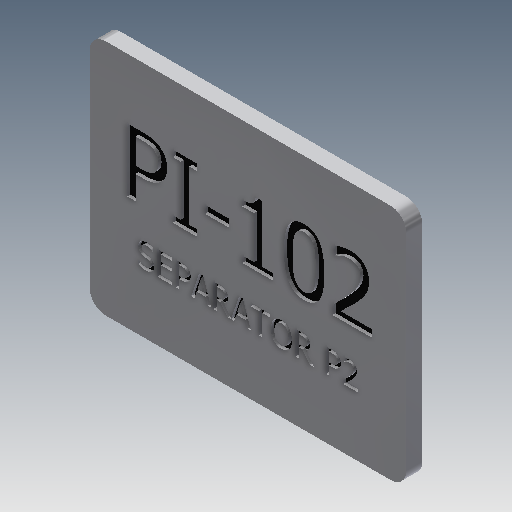
# Autodesk Inventor part: PI-102_Instrument Name Plate
Saved by Autodesk Inventor 2019.1 (Build 231200000, 200)
## iProperties
Created: 2009-08-11
Part Number: PI-102_Instrument Name Plate
Material: Polyaryletherketone Resin
Document SubType Name: Modeling
Designer: Demir Ali
Mass: 48.4669 g
Surface Area: 174.768 cm^2
Volume: 36.7173 cm^3
Density: 1.32 g/cm^3
Description: Name Plate
Stock Number: NA
Appearance: Smooth - White
Title: Purchased Part
Author: Demir Ali
Revision Number: A
Autodesk Inventor part; units mm, degrees
ref_plane "YZ Plane" through (0, 0, 0) normal (1, 0, 0) x (0, 1, 0)
ref_plane "XZ Plane" through (0, 0, 0) normal (0, 1, 0) x (-1, 0, 0)
ref_plane "XY Plane" through (0, 0, 0) normal (0, 0, 1) x (1, 0, 0)
sketch "Sketch1" plane through (0, 0, 0) normal (0, 0, 1) x (1, 0, 0)
  line L0 (-50, -37.5) -> (50, -37.5)
  line L1 (50, -37.5) -> (50, 37.5)
  line L2 (50, 37.5) -> (-50, 37.5)
  line L3 (-50, 37.5) -> (-50, -37.5)
  point P0 (0, 0)
  point P1 (50, 0)
  point P2 (0, 37.5)
  dimension "d0" = 100
  dimension "d1" = 75
  constraints: 8 end point, 2 midpoint, 2 parallel, 1 horizontal, 1 horizontal alignment, 1 perpendicular, 1 vertical alignment
  measures "d0" distance of L1.end L2.end
  measures "d1" distance of L0.end L1.end
extrude "Extrusion1" add sketch "Sketch1" along normal blind 5
sketch "Sketch2" plane through (0, 0, 5) normal (0, 0, 1) x (1, 0, 0)
  line L0 (-39.7109, 33.8079) -> (39.7109, 33.8079) construction
  line L1 (39.7109, 33.8079) -> (39.7109, -33.8079) construction
  line L2 (39.7109, -33.8079) -> (-39.7109, -33.8079) construction
  line L3 (-39.7109, -33.8079) -> (-39.7109, 33.8079) construction
  line L4 (-50, -37.5) -> (-50, 37.5) projected
  line L5 (50, -37.5) -> (-50, -37.5) projected
  line L6 (50, 37.5) -> (50, -37.5) projected
  line L7 (-50, 37.5) -> (50, 37.5) projected
  spline S0 degree 2 poles (-25.5511, 12.4253) (-25.5511, 11.1287) (-26.4749, 8.7948) (-27.3015, 7.9844) knots 0 0 0 1 2 2 2
  spline S1 degree 2 poles (-27.3015, 7.9844) (-28.3387, 6.9633) (-31.1426, 5.9099) (-33.282, 5.9099) knots 0 0 0 1 2 2 2
  line L8 (-33.282, 5.9099) -> (-35.5348, 5.9099)
  line L9 (-35.5348, 5.9099) -> (-35.5348, -1.5456)
  line L10 (-35.5348, -1.5456) -> (-38.1929, -1.5456)
  line L11 (-38.1929, -1.5456) -> (-38.1929, 18.4544)
  line L12 (-38.1929, 18.4544) -> (-33.1686, 18.4544)
  spline S2 degree 2 poles (-33.1686, 18.4544) (-31.3857, 18.4544) (-28.8898, 17.871) (-27.9336, 17.2065) knots 0 0 0 1 2 2 2
  spline S3 degree 2 poles (-27.9336, 17.2065) (-26.8152, 16.4447) (-25.5511, 14.0946) (-25.5511, 12.4253) knots 0 0 0 1 2 2 2
  spline S4 degree 2 poles (-28.3225, 12.3442) (-28.3225, 13.3815) (-29.0357, 14.905) (-29.765, 15.3912) knots 0 0 0 1 2 2 2
  spline S5 degree 2 poles (-29.765, 15.3912) (-30.3971, 15.8126) (-32.0827, 16.153) (-33.3306, 16.153) knots 0 0 0 1 2 2 2
  line L13 (-33.3306, 16.153) -> (-35.5348, 16.153)
  line L14 (-35.5348, 16.153) -> (-35.5348, 8.1789)
  line L15 (-35.5348, 8.1789) -> (-33.7196, 8.1789)
  spline S6 degree 2 poles (-33.7196, 8.1789) (-32.0989, 8.1789) (-30.1053, 8.6975) (-29.4571, 9.3783) knots 0 0 0 1 2 2 2
  spline S7 degree 2 poles (-29.4571, 9.3783) (-28.8574, 9.9779) (-28.3225, 11.388) (-28.3225, 12.3442) knots 0 0 0 1 2 2 2
  line L16 (-16.0535, -1.5456) -> (-23.8006, -1.5456)
  line L17 (-23.8006, -1.5456) -> (-23.8006, 0.4966)
  line L18 (-23.8006, 0.4966) -> (-21.2561, 0.4966)
  line L19 (-21.2561, 0.4966) -> (-21.2561, 16.4123)
  line L20 (-21.2561, 16.4123) -> (-23.8006, 16.4123)
  line L21 (-23.8006, 16.4123) -> (-23.8006, 18.4544)
  line L22 (-23.8006, 18.4544) -> (-16.0535, 18.4544)
  line L23 (-16.0535, 18.4544) -> (-16.0535, 16.4123)
  line L24 (-16.0535, 16.4123) -> (-18.5981, 16.4123)
  line L25 (-18.5981, 16.4123) -> (-18.5981, 0.4966)
  line L26 (-18.5981, 0.4966) -> (-16.0535, 0.4966)
  line L27 (-16.0535, 0.4966) -> (-16.0535, -1.5456)
  line L28 (-6.0049, 5.9909) -> (-13.5737, 5.9909)
  line L29 (-13.5737, 5.9909) -> (-13.5737, 8.422)
  line L30 (-13.5737, 8.422) -> (-6.0049, 8.422)
  line L31 (-6.0049, 8.422) -> (-6.0049, 5.9909)
  line L32 (7.9822, -1.5456) -> (-1.7747, -1.5456)
  line L33 (-1.7747, -1.5456) -> (-1.7747, 0.4966)
  line L34 (-1.7747, 0.4966) -> (1.8558, 0.4966)
  line L35 (1.8558, 0.4966) -> (1.8558, 13.9001)
  line L36 (1.8558, 13.9001) -> (-1.7747, 13.9001)
  line L37 (-1.7747, 13.9001) -> (-1.7747, 15.7316)
  spline S8 degree 2 poles (-1.7747, 15.7316) (0.2836, 15.7316) (2.2285, 16.8985) (2.3582, 18.5193) knots 0 0 0 1 2 2 2
  line L38 (2.3582, 18.5193) -> (4.4327, 18.5193)
  line L39 (4.4327, 18.5193) -> (4.4327, 0.4966)
  line L40 (4.4327, 0.4966) -> (7.9822, 0.4966)
  line L41 (7.9822, 0.4966) -> (7.9822, -1.5456)
  spline S9 degree 2 poles (24.1086, 8.4544) (24.1086, 3.0736) (20.9806, -1.967) (17.7229, -1.967) knots 0 0 0 1 2 2 2
  spline S10 degree 2 poles (17.7229, -1.967) (14.4165, -1.967) (11.3209, 3.1708) (11.3209, 8.4382) knots 0 0 0 1 2 2 2
  spline S11 degree 2 poles (11.3209, 8.4382) (11.3209, 13.8515) (14.4489, 18.8596) (17.7229, 18.8596) knots 0 0 0 1 2 2 2
  spline S12 degree 2 poles (17.7229, 18.8596) (21.013, 18.8596) (24.1086, 13.6732) (24.1086, 8.4544) knots 0 0 0 1 2 2 2
  spline S13 degree 2 poles (20.6726, 2.3604) (21.0616, 3.3491) (21.3857, 6.3961) (21.3857, 8.4544) knots 0 0 0 1 2 2 2
  spline S14 degree 2 poles (21.3857, 8.4544) (21.3857, 10.5128) (21.0616, 13.5436) (20.6564, 14.5646) knots 0 0 0 1 2 2 2
  spline S15 degree 2 poles (20.6564, 14.5646) (20.2512, 15.5857) (18.8412, 16.6392) (17.7229, 16.6392) knots 0 0 0 1 2 2 2
  spline S16 degree 2 poles (17.7229, 16.6392) (16.6045, 16.6392) (15.1621, 15.5857) (14.7407, 14.5322) knots 0 0 0 1 2 2 2
  spline S17 degree 2 poles (14.7407, 14.5322) (14.3355, 13.5112) (14.0438, 10.3993) (14.0438, 8.4382) knots 0 0 0 1 2 2 2
  spline S18 degree 2 poles (14.0438, 8.4382) (14.0438, 6.3313) (14.3031, 3.5112) (14.7245, 2.4091) knots 0 0 0 1 2 2 2
  spline S19 degree 2 poles (14.7245, 2.4091) (15.1135, 1.3718) (16.5559, 0.2535) (17.7229, 0.2535) knots 0 0 0 1 2 2 2
  spline S20 degree 2 poles (17.7229, 0.2535) (18.825, 0.2535) (20.2674, 1.3069) (20.6726, 2.3604) knots 0 0 0 1 2 2 2
  line L42 (39.0032, -1.5456) -> (26.6694, -1.5456)
  line L43 (26.6694, -1.5456) -> (26.6694, 1.2907)
  spline S21 degree 2 poles (26.6694, 1.2907) (27.9984, 2.5387) (30.3647, 4.8564) (31.4992, 6.1044) knots 0 0 0 1 2 2 2
  spline S22 degree 2 poles (31.4992, 6.1044) (33.7844, 8.6165) (35.4538, 11.6311) (35.4538, 13.2356) knots 0 0 0 1 2 2 2
  spline S23 degree 2 poles (35.4538, 13.2356) (35.4538, 14.0784) (34.9352, 15.3426) (34.4652, 15.7478) knots 0 0 0 1 2 2 2
  spline S24 degree 2 poles (34.4652, 15.7478) (33.9951, 16.153) (32.7634, 16.5582) (32.0178, 16.5582) knots 0 0 0 1 2 2 2
  spline S25 degree 2 poles (32.0178, 16.5582) (31.3047, 16.5582) (29.846, 16.2016) (29.1815, 15.9261) knots 0 0 0 1 2 2 2
  spline S26 degree 2 poles (29.1815, 15.9261) (28.6143, 15.6992) (27.5608, 15.0509) (27.2366, 14.824) knots 0 0 0 1 2 2 2
  line L44 (27.2366, 14.824) -> (27.0908, 14.824)
  line L45 (27.0908, 14.824) -> (27.0908, 17.6765)
  spline S27 degree 2 poles (27.0908, 17.6765) (27.9173, 18.0817) (30.8833, 18.8758) (32.2123, 18.8758) knots 0 0 0 1 2 2 2
  spline S28 degree 2 poles (32.2123, 18.8758) (35.0162, 18.8758) (38.1767, 15.9099) (38.1767, 13.3815) knots 0 0 0 1 2 2 2
  spline S29 degree 2 poles (38.1767, 13.3815) (38.1767, 12.1984) (37.6256, 10.221) (37.1394, 9.3783) knots 0 0 0 1 2 2 2
  spline S30 degree 2 poles (37.1394, 9.3783) (36.6532, 8.5031) (35.2431, 6.7851) (34.4652, 5.9585) knots 0 0 0 1 2 2 2
  spline S31 degree 2 poles (34.4652, 5.9585) (33.201, 4.5809) (30.1053, 1.6311) (29.1815, 0.7721) knots 0 0 0 1 2 2 2
  line L46 (29.1815, 0.7721) -> (39.0032, 0.7721)
  line L47 (39.0032, 0.7721) -> (39.0032, -1.5456)
  spline S32 degree 2 poles (-32.2761, -18.8515) (-33.0906, -18.8515) (-34.2332, -18.5112) (-34.7376, -18.268) knots 0 0 0 1 2 2 2
  line L48 (-34.7376, -18.268) -> (-34.7376, -17.016)
  line L49 (-34.7376, -17.016) -> (-34.6647, -17.016)
  spline S33 degree 2 poles (-34.6647, -17.016) (-34.1724, -17.4779) (-32.9265, -17.9885) (-32.3491, -17.9885) knots 0 0 0 1 2 2 2
  spline S34 degree 2 poles (-32.3491, -17.9885) (-31.5225, -17.9885) (-30.6777, -17.3017) (-30.6777, -16.7364) knots 0 0 0 1 2 2 2
  spline S35 degree 2 poles (-30.6777, -16.7364) (-30.6777, -16.2867) (-31.1214, -15.7275) (-31.6015, -15.5877) knots 0 0 0 1 2 2 2
  spline S36 degree 2 poles (-31.6015, -15.5877) (-31.9479, -15.4905) (-32.5253, -15.3568) (-32.9568, -15.2474) knots 0 0 0 1 2 2 2
  spline S37 degree 2 poles (-32.9568, -15.2474) (-33.3458, -15.1441) (-33.9597, -14.8341) (-34.1967, -14.5849) knots 0 0 0 1 2 2 2
  spline S38 degree 2 poles (-34.1967, -14.5849) (-34.4277, -14.3357) (-34.6829, -13.6672) (-34.6829, -13.2296) knots 0 0 0 1 2 2 2
  spline S39 degree 2 poles (-34.6829, -13.2296) (-34.6829, -12.3179) (-33.2607, -11.0841) (-32.1607, -11.0841) knots 0 0 0 1 2 2 2
  spline S40 degree 2 poles (-32.1607, -11.0841) (-31.5286, -11.0841) (-30.4103, -11.3333) (-29.9301, -11.5703) knots 0 0 0 1 2 2 2
  line L50 (-29.9301, -11.5703) -> (-29.9301, -12.7616)
  line L51 (-29.9301, -12.7616) -> (-30.003, -12.7616)
  spline S41 degree 2 poles (-30.003, -12.7616) (-30.3616, -12.4334) (-31.4799, -11.9471) (-32.0938, -11.9471) knots 0 0 0 1 2 2 2
  spline S42 degree 2 poles (-32.0938, -11.9471) (-32.7867, -11.9471) (-33.6436, -12.5975) (-33.6436, -13.1262) knots 0 0 0 1 2 2 2
  spline S43 degree 2 poles (-33.6436, -13.1262) (-33.6436, -13.6003) (-33.1392, -14.1655) (-32.6651, -14.2932) knots 0 0 0 1 2 2 2
  spline S44 degree 2 poles (-32.6651, -14.2932) (-32.3491, -14.3783) (-31.4313, -14.5971) (-31.1274, -14.6882) knots 0 0 0 1 2 2 2
  spline S45 degree 2 poles (-31.1274, -14.6882) (-30.3556, -14.9253) (-29.6384, -15.8795) (-29.6384, -16.5784) knots 0 0 0 1 2 2 2
  spline S46 degree 2 poles (-29.6384, -16.5784) (-29.6384, -17.0221) (-29.997, -17.873) (-30.3191, -18.1708) knots 0 0 0 1 2 2 2
  spline S47 degree 2 poles (-30.3191, -18.1708) (-30.6777, -18.499) (-31.5893, -18.8515) (-32.2761, -18.8515) knots 0 0 0 1 2 2 2
  line L52 (-28.6234, -18.7178) -> (-28.6234, -11.2178)
  line L53 (-28.6234, -11.2178) -> (-23.9313, -11.2178)
  line L54 (-23.9313, -11.2178) -> (-23.9313, -12.1052)
  line L55 (-23.9313, -12.1052) -> (-27.6266, -12.1052)
  line L56 (-27.6266, -12.1052) -> (-27.6266, -14.1595)
  line L57 (-27.6266, -14.1595) -> (-24.1805, -14.1595)
  line L58 (-24.1805, -14.1595) -> (-24.1805, -15.0468)
  line L59 (-24.1805, -15.0468) -> (-27.6266, -15.0468)
  line L60 (-27.6266, -15.0468) -> (-27.6266, -17.8304)
  line L61 (-27.6266, -17.8304) -> (-23.9313, -17.8304)
  line L62 (-23.9313, -17.8304) -> (-23.9313, -18.7178)
  line L63 (-23.9313, -18.7178) -> (-28.6234, -18.7178)
  spline S48 degree 2 poles (-18.0966, -13.4787) (-18.0966, -13.965) (-18.4431, -14.8402) (-18.753, -15.1441) knots 0 0 0 1 2 2 2
  spline S49 degree 2 poles (-18.753, -15.1441) (-19.142, -15.527) (-20.1935, -15.922) (-20.9957, -15.922) knots 0 0 0 1 2 2 2
  line L64 (-20.9957, -15.922) -> (-21.8406, -15.922)
  line L65 (-21.8406, -15.922) -> (-21.8406, -18.7178)
  line L66 (-21.8406, -18.7178) -> (-22.8373, -18.7178)
  line L67 (-22.8373, -18.7178) -> (-22.8373, -11.2178)
  line L68 (-22.8373, -11.2178) -> (-20.9532, -11.2178)
  spline S50 degree 2 poles (-20.9532, -11.2178) (-20.2846, -11.2178) (-19.3487, -11.4366) (-18.9901, -11.6858) knots 0 0 0 1 2 2 2
  spline S51 degree 2 poles (-18.9901, -11.6858) (-18.5707, -11.9714) (-18.0966, -12.8527) (-18.0966, -13.4787) knots 0 0 0 1 2 2 2
  spline S52 degree 2 poles (-19.1359, -13.5091) (-19.1359, -13.1202) (-19.4034, -12.5488) (-19.6769, -12.3665) knots 0 0 0 1 2 2 2
  spline S53 degree 2 poles (-19.6769, -12.3665) (-19.9139, -12.2085) (-20.546, -12.0808) (-21.014, -12.0808) knots 0 0 0 1 2 2 2
  line L69 (-21.014, -12.0808) -> (-21.8406, -12.0808)
  line L70 (-21.8406, -12.0808) -> (-21.8406, -15.0711)
  line L71 (-21.8406, -15.0711) -> (-21.1598, -15.0711)
  spline S54 degree 2 poles (-21.1598, -15.0711) (-20.5521, -15.0711) (-19.8045, -14.8766) (-19.5614, -14.6214) knots 0 0 0 1 2 2 2
  spline S55 degree 2 poles (-19.5614, -14.6214) (-19.3365, -14.3965) (-19.1359, -13.8677) (-19.1359, -13.5091) knots 0 0 0 1 2 2 2
  line L72 (-17.9568, -18.7178) -> (-15.4285, -11.2178)
  line L73 (-15.4285, -11.2178) -> (-14.2008, -11.2178)
  line L74 (-14.2008, -11.2178) -> (-11.6724, -18.7178)
  line L75 (-11.6724, -18.7178) -> (-12.7239, -18.7178)
  line L76 (-12.7239, -18.7178) -> (-13.4046, -16.621)
  line L77 (-13.4046, -16.621) -> (-16.2672, -16.621)
  line L78 (-16.2672, -16.621) -> (-16.9479, -18.7178)
  line L79 (-16.9479, -18.7178) -> (-17.9568, -18.7178)
  line L80 (-13.6781, -15.7701) -> (-14.8389, -12.2389)
  line L81 (-14.8389, -12.2389) -> (-15.9937, -15.7701)
  line L82 (-15.9937, -15.7701) -> (-13.6781, -15.7701)
  line L83 (-5.157, -18.7178) -> (-6.4516, -18.7178)
  line L84 (-6.4516, -18.7178) -> (-8.8219, -15.7336)
  line L85 (-8.8219, -15.7336) -> (-9.9645, -15.7336)
  line L86 (-9.9645, -15.7336) -> (-9.9645, -18.7178)
  line L87 (-9.9645, -18.7178) -> (-10.9613, -18.7178)
  line L88 (-10.9613, -18.7178) -> (-10.9613, -11.2178)
  line L89 (-10.9613, -11.2178) -> (-9.0286, -11.2178)
  spline S56 degree 2 poles (-9.0286, -11.2178) (-8.3843, -11.2178) (-7.5152, -11.3576) (-7.1201, -11.6129) knots 0 0 0 1 2 2 2
  spline S57 degree 2 poles (-7.1201, -11.6129) (-6.7251, -11.8681) (-6.2692, -12.6643) (-6.2692, -13.2539) knots 0 0 0 1 2 2 2
  spline S58 degree 2 poles (-6.2692, -13.2539) (-6.2692, -14.0744) (-7.108, -15.1866) (-7.8252, -15.454) knots 0 0 0 1 2 2 2
  line L90 (-7.8252, -15.454) -> (-5.157, -18.7178)
  spline S59 degree 2 poles (-7.3086, -13.3329) (-7.3086, -13.0047) (-7.5395, -12.5002) (-7.7826, -12.3361) knots 0 0 0 1 2 2 2
  spline S60 degree 2 poles (-7.7826, -12.3361) (-7.9953, -12.1963) (-8.5606, -12.0808) (-8.9739, -12.0808) knots 0 0 0 1 2 2 2
  line L91 (-8.9739, -12.0808) -> (-9.9645, -12.0808)
  line L92 (-9.9645, -12.0808) -> (-9.9645, -14.9009)
  line L93 (-9.9645, -14.9009) -> (-9.0893, -14.9009)
  spline S61 degree 2 poles (-9.0893, -14.9009) (-8.6578, -14.9009) (-7.971, -14.749) (-7.734, -14.512) knots 0 0 0 1 2 2 2
  spline S62 degree 2 poles (-7.734, -14.512) (-7.5152, -14.3053) (-7.3086, -13.7219) (-7.3086, -13.3329) knots 0 0 0 1 2 2 2
  line L94 (-5.3697, -18.7178) -> (-2.8414, -11.2178)
  line L95 (-2.8414, -11.2178) -> (-1.6137, -11.2178)
  line L96 (-1.6137, -11.2178) -> (0.9147, -18.7178)
  line L97 (0.9147, -18.7178) -> (-0.1368, -18.7178)
  line L98 (-0.1368, -18.7178) -> (-0.8175, -16.621)
  line L99 (-0.8175, -16.621) -> (-3.6801, -16.621)
  line L100 (-3.6801, -16.621) -> (-4.3608, -18.7178)
  line L101 (-4.3608, -18.7178) -> (-5.3697, -18.7178)
  line L102 (-1.091, -15.7701) -> (-2.2518, -12.2389)
  line L103 (-2.2518, -12.2389) -> (-3.4066, -15.7701)
  line L104 (-3.4066, -15.7701) -> (-1.091, -15.7701)
  line L105 (3.3762, -18.7178) -> (3.3762, -12.1052)
  line L106 (3.3762, -12.1052) -> (0.86, -12.1052)
  line L107 (0.86, -12.1052) -> (0.86, -11.2178)
  line L108 (0.86, -11.2178) -> (6.8892, -11.2178)
  line L109 (6.8892, -11.2178) -> (6.8892, -12.1052)
  line L110 (6.8892, -12.1052) -> (4.373, -12.1052)
  line L111 (4.373, -12.1052) -> (4.373, -18.7178)
  line L112 (4.373, -18.7178) -> (3.3762, -18.7178)
  spline S63 degree 2 poles (12.9548, -12.0748) (13.3803, -12.5732) (13.8543, -14.0318) (13.8543, -14.9678) knots 0 0 0 1 2 2 2
  spline S64 degree 2 poles (13.8543, -14.9678) (13.8543, -15.8795) (13.3924, -17.3564) (12.9548, -17.8548) knots 0 0 0 1 2 2 2
  spline S65 degree 2 poles (12.9548, -17.8548) (12.4929, -18.3774) (11.2713, -18.8758) (10.5359, -18.8758) knots 0 0 0 1 2 2 2
  spline S66 degree 2 poles (10.5359, -18.8758) (9.7761, -18.8758) (8.5606, -18.3592) (8.1169, -17.8548) knots 0 0 0 1 2 2 2
  spline S67 degree 2 poles (8.1169, -17.8548) (7.6854, -17.3564) (7.2235, -15.8916) (7.2235, -14.9678) knots 0 0 0 1 2 2 2
  spline S68 degree 2 poles (7.2235, -14.9678) (7.2235, -14.0257) (7.6914, -12.5914) (8.123, -12.0748) knots 0 0 0 1 2 2 2
  spline S69 degree 2 poles (8.123, -12.0748) (8.5606, -11.5764) (9.7822, -11.0598) (10.5359, -11.0598) knots 0 0 0 1 2 2 2
  spline S70 degree 2 poles (10.5359, -11.0598) (11.3017, -11.0598) (12.5294, -11.5946) (12.9548, -12.0748) knots 0 0 0 1 2 2 2
  spline S71 degree 2 poles (12.815, -14.9678) (12.815, -14.2263) (12.4929, -13.0776) (12.2012, -12.7008) knots 0 0 0 1 2 2 2
  spline S72 degree 2 poles (12.2012, -12.7008) (11.9034, -12.3118) (11.0646, -11.9228) (10.5419, -11.9228) knots 0 0 0 1 2 2 2
  spline S73 degree 2 poles (10.5419, -11.9228) (10.001, -11.9228) (9.1866, -12.2997) (8.8766, -12.7008) knots 0 0 0 1 2 2 2
  spline S74 degree 2 poles (8.8766, -12.7008) (8.5788, -13.0837) (8.2628, -14.2385) (8.2628, -14.9678) knots 0 0 0 1 2 2 2
  spline S75 degree 2 poles (8.2628, -14.9678) (8.2628, -16.4447) (9.5026, -18.0128) (10.5419, -18.0128) knots 0 0 0 1 2 2 2
  spline S76 degree 2 poles (10.5419, -18.0128) (11.5812, -18.0128) (12.815, -16.4447) (12.815, -14.9678) knots 0 0 0 1 2 2 2
  line L113 (20.7526, -18.7178) -> (19.4581, -18.7178)
  line L114 (19.4581, -18.7178) -> (17.0877, -15.7336)
  line L115 (17.0877, -15.7336) -> (15.9451, -15.7336)
  line L116 (15.9451, -15.7336) -> (15.9451, -18.7178)
  line L117 (15.9451, -18.7178) -> (14.9483, -18.7178)
  line L118 (14.9483, -18.7178) -> (14.9483, -11.2178)
  line L119 (14.9483, -11.2178) -> (16.8811, -11.2178)
  spline S77 degree 2 poles (16.8811, -11.2178) (17.5253, -11.2178) (18.3944, -11.3576) (18.7895, -11.6129) knots 0 0 0 1 2 2 2
  spline S78 degree 2 poles (18.7895, -11.6129) (19.1846, -11.8681) (19.6404, -12.6643) (19.6404, -13.2539) knots 0 0 0 1 2 2 2
  spline S79 degree 2 poles (19.6404, -13.2539) (19.6404, -14.0744) (18.8017, -15.1866) (18.0845, -15.454) knots 0 0 0 1 2 2 2
  line L120 (18.0845, -15.454) -> (20.7526, -18.7178)
  spline S80 degree 2 poles (18.6011, -13.3329) (18.6011, -13.0047) (18.3701, -12.5002) (18.127, -12.3361) knots 0 0 0 1 2 2 2
  spline S81 degree 2 poles (18.127, -12.3361) (17.9143, -12.1963) (17.3491, -12.0808) (16.9358, -12.0808) knots 0 0 0 1 2 2 2
  line L121 (16.9358, -12.0808) -> (15.9451, -12.0808)
  line L122 (15.9451, -12.0808) -> (15.9451, -14.9009)
  line L123 (15.9451, -14.9009) -> (16.8203, -14.9009)
  spline S82 degree 2 poles (16.8203, -14.9009) (17.2518, -14.9009) (17.9386, -14.749) (18.1756, -14.512) knots 0 0 0 1 2 2 2
  spline S83 degree 2 poles (18.1756, -14.512) (18.3944, -14.3053) (18.6011, -13.7219) (18.6011, -13.3329) knots 0 0 0 1 2 2 2
  spline S84 degree 2 poles (29.3102, -13.4787) (29.3102, -13.965) (28.9637, -14.8402) (28.6538, -15.1441) knots 0 0 0 1 2 2 2
  spline S85 degree 2 poles (28.6538, -15.1441) (28.2648, -15.527) (27.2133, -15.922) (26.4111, -15.922) knots 0 0 0 1 2 2 2
  line L124 (26.4111, -15.922) -> (25.5662, -15.922)
  line L125 (25.5662, -15.922) -> (25.5662, -18.7178)
  line L126 (25.5662, -18.7178) -> (24.5695, -18.7178)
  line L127 (24.5695, -18.7178) -> (24.5695, -11.2178)
  line L128 (24.5695, -11.2178) -> (26.4536, -11.2178)
  spline S86 degree 2 poles (26.4536, -11.2178) (27.1222, -11.2178) (28.0581, -11.4366) (28.4167, -11.6858) knots 0 0 0 1 2 2 2
  spline S87 degree 2 poles (28.4167, -11.6858) (28.8361, -11.9714) (29.3102, -12.8527) (29.3102, -13.4787) knots 0 0 0 1 2 2 2
  spline S88 degree 2 poles (28.2709, -13.5091) (28.2709, -13.1202) (28.0034, -12.5488) (27.7299, -12.3665) knots 0 0 0 1 2 2 2
  spline S89 degree 2 poles (27.7299, -12.3665) (27.4929, -12.2085) (26.8608, -12.0808) (26.3928, -12.0808) knots 0 0 0 1 2 2 2
  line L129 (26.3928, -12.0808) -> (25.5662, -12.0808)
  line L130 (25.5662, -12.0808) -> (25.5662, -15.0711)
  line L131 (25.5662, -15.0711) -> (26.247, -15.0711)
  spline S90 degree 2 poles (26.247, -15.0711) (26.8547, -15.0711) (27.6023, -14.8766) (27.8454, -14.6214) knots 0 0 0 1 2 2 2
  spline S91 degree 2 poles (27.8454, -14.6214) (28.0703, -14.3965) (28.2709, -13.8677) (28.2709, -13.5091) knots 0 0 0 1 2 2 2
  line L132 (34.6708, -18.7178) -> (30.0456, -18.7178)
  line L133 (30.0456, -18.7178) -> (30.0456, -17.6542)
  spline S92 degree 2 poles (30.0456, -17.6542) (30.544, -17.1862) (31.4313, -16.3171) (31.8568, -15.8491) knots 0 0 0 1 2 2 2
  spline S93 degree 2 poles (31.8568, -15.8491) (32.7137, -14.907) (33.3397, -13.7766) (33.3397, -13.1749) knots 0 0 0 1 2 2 2
  spline S94 degree 2 poles (33.3397, -13.1749) (33.3397, -12.8588) (33.1453, -12.3847) (32.969, -12.2328) knots 0 0 0 1 2 2 2
  spline S95 degree 2 poles (32.969, -12.2328) (32.7927, -12.0808) (32.3308, -11.9289) (32.0513, -11.9289) knots 0 0 0 1 2 2 2
  spline S96 degree 2 poles (32.0513, -11.9289) (31.7838, -11.9289) (31.2368, -12.0626) (30.9876, -12.1659) knots 0 0 0 1 2 2 2
  spline S97 degree 2 poles (30.9876, -12.1659) (30.7749, -12.251) (30.3799, -12.4941) (30.2583, -12.5792) knots 0 0 0 1 2 2 2
  line L134 (30.2583, -12.5792) -> (30.2036, -12.5792)
  line L135 (30.2036, -12.5792) -> (30.2036, -11.5095)
  spline S98 degree 2 poles (30.2036, -11.5095) (30.5136, -11.3576) (31.6258, -11.0598) (32.1242, -11.0598) knots 0 0 0 1 2 2 2
  spline S99 degree 2 poles (32.1242, -11.0598) (33.1756, -11.0598) (34.3608, -12.172) (34.3608, -13.1202) knots 0 0 0 1 2 2 2
  spline S100 degree 2 poles (34.3608, -13.1202) (34.3608, -13.5638) (34.1542, -14.3053) (33.9718, -14.6214) knots 0 0 0 1 2 2 2
  spline S101 degree 2 poles (33.9718, -14.6214) (33.7895, -14.9496) (33.2607, -15.5938) (32.969, -15.9038) knots 0 0 0 1 2 2 2
  spline S102 degree 2 poles (32.969, -15.9038) (32.4949, -16.4204) (31.3341, -17.5266) (30.9876, -17.8487) knots 0 0 0 1 2 2 2
  line L136 (30.9876, -17.8487) -> (34.6708, -17.8487)
  line L137 (34.6708, -17.8487) -> (34.6708, -18.7178)
  point P0 (0, 0)
  point P1 (0, 33.8079)
  point P2 (-39.7109, 0)
  constraints: 2 midpoint, 1 horizontal alignment, 1 vertical alignment, 2 other
emboss "Emboss1" sketch "Sketch2" operation cut depth 1 direction (0, 0, -1) contours S0 S1 L8 L9 L10 L11 L12 S2 S3 | L16 L17 L18 L19 L20 L21 L22 L23 L24 L25 L26 L27 | L28 L29 L30 L31 | L32 L33 L34 L35 L36 L37 S8 L38 L39 L40 L41 | S9 S10 S11 S12 | L42 L43 S21 S22 S23 S24 S25 S26 L44 L45 S27 S28 S29 S30 S31 L46 L47 | S32 L48 L49 S33 S34 S35 S36 S37 S38 S39 S40 L50 L51 S41 S42 S43 S44 S45 S46 S47 | L52 L53 L54 L55 L56 L57 L58 L59 L60 L61 L62 L63 | S48 S49 L64 L65 L66 L67 L68 S50 S51 | L72 L73 L74 L75 L76 L77 L78 L79 | L83 L94 L90 | L90 L94 L95 L96 L97 L98 L99 L100 L101 | L83 L84 L85 L86 L87 L88 L89 S56 S57 S58 L90 L94 | L105 L106 L107 L108 L109 L110 L111 L112 | S63 S64 S65 S66 S67 S68 S69 S70 | L113 L114 L115 L116 L117 L118 L119 S77 S78 S79 L120 | S84 S85 L124 L125 L126 L127 L128 S86 S87 | L132 L133 S92 S93 S94 S95 S96 S97 L134 L135 S98 S99 S100 S101 S102 L136 L137
fillet "Fillet1" radius 5 4 edges at (-50, 37.5, 2.5) (50, 37.5, 2.5) (-50, -37.5, 2.5) (50, -37.5, 2.5)
body "Solid1"
